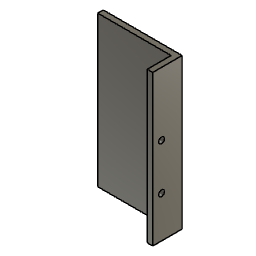
오린 브라켓 (Autodesk Fusion 360 design; units mm, degrees)
Autodesk Fusion 360 part; units mm, degrees
note: some values were not read from the file. Set by a fixed rule: which sketch regions a step uses.
sketch "스케치1" plane through (0, 0, 0) normal (1, 0, 0) x (0, 1, 0)
  line L0 (0, 0) -> (-16, 0)
  line L1 (-16, 0) -> (-16, 82)
  line L2 (-16, 82) -> (0, 82)
  line L3 (0, 82) -> (0, 0)
  line L4 (0, 0) -> (-6, 0)
  line L5 (-6, 0) -> (-6, 82)
  line L6 (-6, 82) -> (0, 82)
  line L7 (0, 82) -> (0, 0)
  line L8 (-6, 0) -> (-11.2, 0)
  line L9 (-11.2, 0) -> (-11.2, 22.5)
  line L10 (-11.2, 22.5) -> (-6, 22.5)
  line L11 (-6, 22.5) -> (-6, 0)
  circle A0 centre (-11.2, 22.5) radius 1.6
  line L12 (-11.2, 22.5) -> (-11.2, 47.5)
  circle A1 centre (-11.2, 47.5) radius 1.6
  line L13 (0, 0) -> (-3, 0)
  line L14 (-3, 0) -> (-3, 82)
  line L15 (-3, 82) -> (0, 82)
  line L16 (0, 82) -> (0, 0)
  dimension "d1" = 16
  dimension "d2" = 82
  dimension "d3" = 6
  dimension "d4" = 82
  dimension "d5" = 5.2
  dimension "d6" = 22.5
  dimension "d7" = 3.2
  dimension "d8" = 25
  dimension "d9" = 3.2
  dimension "d14" = 3
  dimension "d15" = 82
  constraint horizontal L0
  constraint vertical L1
  constraint horizontal L2
  constraint vertical L3
  constraint coincident L0.start L3.end
  constraint horizontal L4
  constraint vertical L5
  constraint horizontal L6
  constraint vertical L7
  constraint horizontal L8
  constraint vertical L9
  constraint horizontal L10
  constraint vertical L11
  constraint coincident L9.end L10.start
  constraint perpendicular L10 L12
  constraint coincident L12.end A1.centre
  constraint horizontal L13
  constraint vertical L14
  constraint horizontal L15
  constraint vertical L16
  measures "d1" distance of L0.start L0.end
  measures "d2" distance of L0.start L2.end
  measures "d3" distance of L0.start L4.end
  measures "d4" distance of L0.start L2.end
  measures "d5" distance of L4.end L8.end
  measures "d6" distance of L4.end L10.end
  measures "d7" diameter of A0
  measures "d8" distance of L9.end L12.end
  measures "d9" diameter of A1
  measures "d14" distance of L0.start L13.end
  measures "d15" distance of L0.start L2.end
extrude "돌출1" add sketch "스케치1" along normal blind 3 contours L0 L5 L8 L9 L10 L11 A0 | L0 L1 L2 L5 L9 L10 A0
extrude "돌출2" add sketch "스케치1" along normal blind 3 contours L0 L2 L3 L4 L6 L7 L13 L14 L15 L16 | L0 L2 L4 L5 L6 L11 L14
extrude "돌출3" add sketch "스케치1" against normal blind 40 contours L0 L2 L3 L4 L6 L7 L13 L14 L15 L16
